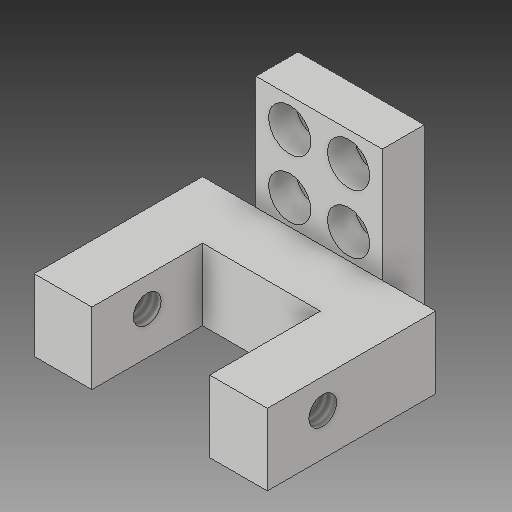
# Autodesk Inventor part: Sample holder long L_V4
Saved by Autodesk Inventor 2019 (Build 230136000, 136)
## iProperties
Created: 2018-08-28
Part Number: Sample holder long L_V4
Material: Generic
Document SubType Name: Sheet Metal
Designer: FiolkaLab
Density: 1 g/cm^3
Sheet Metal Rule: Default_mm
Appearance: Default
Author: FiolkaLab
Autodesk Inventor part; units mm, degrees
ref_plane "YZ Plane" through (0, 0, 0) normal (1, 0, 0) x (0, 1, 0)
ref_plane "XZ Plane" through (0, 0, 0) normal (0, 1, 0) x (-1, 0, 0)
ref_plane "XY Plane" through (0, 0, 0) normal (0, 0, 1) x (1, 0, 0)
sketch "Sketch1" plane through (0, 0, 0) normal (0, 0, 1) x (1, 0, 0)
  line L0 (0, 0) -> (15, 0)
  line L1 (15, 0) -> (15, 22)
  line L2 (15, 22) -> (0, 22)
  line L3 (0, 22) -> (0, 0)
  dimension "d0" = 15
  dimension "d1" = 22
  constraints: 8 end point, 2 parallel, 1 horizontal, 1 perpendicular
  measures "d0" distance of L1.end L2.end
  measures "d1" distance of L0.end L1.end
extrude "Extrusion1" add sketch "Sketch1" along normal blind 5
sketch "Sketch2" plane through (0, 0, 5) normal (0, 0, 1) x (1, 0, 0)
  circle A0 centre (4, 18.5) radius 2.5
  circle A1 centre (11, 18.5) radius 2.5
  circle A2 centre (4, 11.5) radius 2.5
  circle A3 centre (11, 11.5) radius 2.5
  line L0 (15, 22) -> (0, 22) projected
  line L1 (0, 22) -> (0, 0) projected
  line L2 (15, 0) -> (15, 22) projected
  dimension "d4" = 5
  dimension "d5" = 5
  dimension "d6" = 7
  dimension "d7" = 5
  dimension "d8" = 5
  dimension "d9" = 7
  dimension "d10" = 7
  dimension "d11" = 3.5
  dimension "d12" = 3.5
  dimension "d26" = 4
  dimension "d27" = 4
  dimension "d28" = 4
  dimension "d29" = 4
  constraints: 4 centre point
  measures "d4" diameter of A0
  measures "d5" diameter of A1
  measures "d6" distance of A1.centre A0.centre
  measures "d7" diameter of A2
  measures "d8" diameter of A3
  measures "d9" distance of A1.centre A3.centre
  measures "d10" distance of A2.centre A0.centre
  measures "d11" distance from line of L0 A1.centre
  measures "d12" distance from line of L0 A0.centre
  measures "d26" distance from line of L1 A0.centre
  measures "d27" distance from line of L2 A1.centre
  measures "d28" distance from line of L2 A3.centre
  measures "d29" distance from line of L1 A2.centre
hole "Hole1" at (4, 18.5, 5) at (4, 11.5, 5) at (11, 18.5, 5) at (11, 11.5, 5) direction (0, 0, -1) diameter 3.2 end through all counterbore diameter 5 counterbore depth 3.2
sketch "Sketch3" plane through (0, 0, 5) normal (0, 0, 1) x (1, 0, 0)
  line L0 (15, 0) -> (0, 0)
  line L1 (0, 0) -> (0, 8.5)
  line L2 (0, 8.5) -> (15, 8.5)
  line L3 (15, 8.5) -> (15, 0)
  line L4 (15, 0) -> (15, 22) projected
  line L5 (0, 22) -> (0, 0) projected
  line L6 (0, 0) -> (15, 0) projected
  dimension "d20" = 8.5
  dimension "d21" = 0
  dimension "d22" = 0
  dimension "d23" = 0
  constraints: 8 end point, 2 parallel, 1 horizontal, 1 perpendicular
  measures "d20" distance of L2.end L0.start
  measures "d21" distance between parallel lines of L4 L3
  measures "d22" distance between parallel lines of L5 L1
  measures "d23" distance between parallel lines of L6 L0
extrude "Extrusion2" add sketch "Sketch3" along normal blind 20
sketch "Sketch4" plane through (0, 8.5, 5) normal (0, 1, 0) x (1, 0, 0)
  line L0 (0.5, -20) -> (14.5, -20)
  line L1 (14.5, -20) -> (14.5, -6.85)
  line L2 (14.5, -6.85) -> (0.5, -6.85)
  line L3 (0.5, -6.85) -> (0.5, -20)
  line L4 (15, -20) -> (0, -20) projected
  line L5 (0, 0) -> (0, -20) projected
  point P0 (0, 5)
  dimension "d30" = 0
  dimension "d31" = 13.15
  dimension "d32" = 14
  dimension "d33" = 0.5
  constraints: 8 end point, 2 parallel, 1 horizontal, 1 perpendicular
  measures "d30" distance between parallel lines of L4 L0
  measures "d31" distance of L0.end L1.end
  measures "d32" distance of L0.start L0.end
  measures "d33" distance between parallel lines of L5 L3
extrude "Extrusion3" cut sketch "Sketch4" against normal blind 8.5
sketch "Sketch6" plane through (0.5, 8.5, 25) normal (1, 0, 0) x (0, 0, -1)
  circle A0 centre (6.575, -3.5) radius 1.5
  line L0 (0, 0) -> (13.15, 0) projected
  line L1 (0, -8.5) -> (0, 0) projected
  point P0 (25, -8.5)
  point P1 (0, -7)
  dimension "d42" = 3
  dimension "d43" = 3.5
  dimension "d44" = 6.575
  dimension "d83" = 13.15
  dimension "d84" = 7
  constraints: 1 centre point
  measures "d42" diameter of A0
  measures "d43" distance from line of L0 A0.centre
  measures "d44" distance from line of L1 A0.centre
  measures "d83" distance of L0.start L0.end
  measures "d84" distance of point (0, -7) L0.start
sketch "Sketch7" plane through (14.5, 8.5, 11.85) normal (-1, 0, 0) x (0, 0, 1)
  circle A0 centre (6.575, -3.5) radius 1.5
  line L0 (13.15, 0) -> (13.15, -8.5) projected
  line L1 (0, 0) -> (13.15, 0) projected
  line L2 (0, 0) -> (0, -8.5) projected
  point P0 (-11.85, -8.5)
  point P1 (13.15, -7)
  point P2 (0, -7)
  dimension "d45" = 3
  dimension "d46" = 6.575
  dimension "d47" = 3.5
  dimension "d81" = 13.15
  dimension "d82" = 7
  constraints: 1 centre point
  measures "d45" diameter of A0
  measures "d46" distance from line of L0 A0.centre
  measures "d47" distance from line of L1 A0.centre
  measures "d81" distance between parallel lines of L0 L2
  measures "d82" distance of L0.start point (13.15, -7)
sketch "Sketch8" plane through (15, 0, 0) normal (1, 0, 0) x (0, 0, -1)
  line L0 (0, 0) -> (-25, 0) projected
  line L1 (-5, 8.5) -> (-25, 8.5) projected
  line L2 (-25, 0) -> (-5, 0)
  line L3 (-5, 0) -> (-5, 8.5)
  line L4 (-5, 8.5) -> (-25, 8.5)
  line L5 (-25, 8.5) -> (-25, 0)
  constraints: 8 end point, 2 parallel, 1 horizontal, 1 perpendicular
extrude "Extrusion5" add sketch "Sketch8" along normal blind 6.35
hole "Hole4" at (14.5, 5, 18.425) direction (1, 0, 0) diameter 3.302 end through all thread size "8-32 UNC" class "2B" standard "ANSI Unified Screw Threads"
sketch "Sketch9" plane through (0, 0, 0) normal (-1, 0, 0) x (0, 0, 1)
  line L0 (5, 8.5) -> (25, 8.5) projected
  line L1 (25, 0) -> (5, 0) projected
  line L2 (5, 8.5) -> (25, 8.5)
  line L3 (25, 8.5) -> (25, 0)
  line L4 (25, 0) -> (5, 0)
  line L5 (5, 0) -> (5, 8.5)
  point P0 (0, 0)
  constraints: 8 end point, 2 parallel, 1 horizontal, 1 perpendicular
extrude "Extrusion6" add sketch "Sketch9" along normal blind 6.35
hole "Hole5" at (0.5, 5, 18.425) direction (-1, 0, 0) diameter 3.302 end through all thread size "8-32 UNC" class "2B" standard "ANSI Unified Screw Threads"
equation "\"d5\" = d4"
equation "\"d7\" = d4"
equation "\"d8\" = d4"
equation "\"d12\" = d11"
equation "\"d29\" = d26"
equation "\"d18\" = Thickness"
equation "\"d43\" = 0.5 * d84"
equation "\"d44\" = 0.5 * d83"
equation "\"d46\" = 0.5 * d81"
equation "\"d47\" = 0.5 * d82"
equation "\"BendRadius\" = Thickness"
equation "\"BendReliefWidth\" = Thickness"
equation "\"BendReliefDepth\" = 0.5 * Thickness"
equation "\"CornerReliefSize\" = 4 * Thickness"
equation "\"MinimumRemnant\" = 2 * Thickness"
equation "\"TransitionRadius\" = BendRadius"
equation "\"JacobiRadiusSize\" = BendRadius"
equation "\"GapSize\" = Thickness"
equation "\"Thickness\" = 0.5"
body "Solid1"
